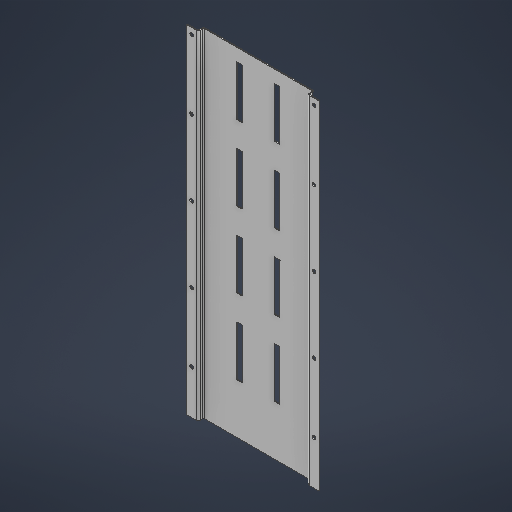
# Autodesk Inventor part: TrayRail
Saved by Autodesk Inventor 2026.3 (Build 303398000, 398)
## iProperties
Created: 2026-05-01
Part Number: TrayRail
Material: Generic
Document SubType Name: Sheet Metal
Designer: frede
Density: 1 g/cm^3
Sheet Metal Rule: Default_mm
Appearance: Default
Author: frede
Autodesk Inventor part; units mm, degrees
ref_plane "YZ Plane" through (0, 0, 0) normal (1, 0, 0) x (0, 1, 0)
ref_plane "XZ Plane" through (0, 0, 0) normal (0, 1, 0) x (-1, 0, 0)
ref_plane "XY Plane" through (0, 0, 0) normal (0, 0, 1) x (1, 0, 0)
sketch "Sketch1" plane through (0, 0, 0) normal (0, 0, 1) x (1, 0, 0)
  line L0 (61, -189) -> (-61, -189)
  line L1 (-61, -189) -> (-61, 189)
  line L2 (-61, 189) -> (61, 189)
  line L3 (61, 189) -> (61, -189)
  line L4 (61, -189) -> (-61, 189) construction
  line L5 (-61, -189) -> (61, 189) construction
  point P0 (0, 0)
  dimension "d0" = 122
  dimension "d1" = 378
  measures "d0" distance of L1.end L2.end
  measures "d1" distance between parallel lines of L0 L2
extrude "Plate1" add sketch "Sketch1" along normal blind 1
sketch "Sketch3" plane through (-62, -189, 0) normal (1, 0, 0) x (0, 1, 0)
  line L0 (378, 0) -> (0, 0)
  line L1 (0, 0) -> (0, 6)
  line L2 (0, 6) -> (378, 6)
  line L3 (378, 6) -> (378, 0)
  constraints: 8 end point
edge flange "Flange1" height 6 angle 90 thickness 1 bend radius 1 thickness toward (1, 0, 0) relief tear relief width 1 relief depth 0.5 corner gap 1 corner form 0 edges at (-61, 0, 1) (61, 0, 1) wall of the first edge with corners at (-62, 189, 0) (-62, -189, 0) (-62, -189, 6) (-62, 189, 6)
bend "Bend1"
corner "Corner1"
sketch "Sketch4" plane through (0, 0, 1) normal (0, 0, 1) x (1, 0, 0)
  line L0 (60, -189) -> (-60, -189) projected
  line L1 (-60, 189) -> (60, 189) projected
  line L2 (60.25, 63) -> (-60.25, 63)
  line L3 (-60.25, 63) -> (-60.25, 189)
  line L4 (-60.25, 189) -> (60.25, 189)
  line L5 (60.25, 189) -> (60.25, 63)
  line L6 (60.25, 63) -> (-60.25, 189) construction
  line L7 (-60.25, 63) -> (60.25, 189) construction
  line L8 (-21, 189) -> (-21, -189)
  line L9 (21, 189) -> (21, -189)
  line L10 (-24.25, 174.5) -> (-24.25, 119.5)
  line L11 (-17.75, 174.5) -> (-17.75, 119.5)
  line L12 (17.75, 174.5) -> (17.75, 119.5)
  line L13 (24.25, 174.5) -> (24.25, 119.5)
  line L14 (-23.75, 175) -> (-18.25, 175)
  line L15 (18.25, 175) -> (23.75, 175)
  line L16 (-23.75, 119) -> (-18.25, 119)
  line L17 (18.25, 119) -> (23.75, 119)
  arc A0 (-23.75, 175) -> (-24.25, 174.5) centre (-23.75, 174.5) ccw
  arc A1 (-17.75, 174.5) -> (-18.25, 175) centre (-18.25, 174.5) ccw
  arc A2 (-18.25, 119) -> (-17.75, 119.5) centre (-18.25, 119.5) ccw
  arc A3 (-24.25, 119.5) -> (-23.75, 119) centre (-23.75, 119.5) ccw
  arc A4 (17.75, 119.5) -> (18.25, 119) centre (18.25, 119.5) ccw
  arc A5 (23.75, 119) -> (24.25, 119.5) centre (23.75, 119.5) ccw
  arc A6 (18.25, 175) -> (17.75, 174.5) centre (18.25, 174.5) ccw
  arc A7 (24.25, 174.5) -> (23.75, 175) centre (23.75, 174.5) ccw
  line L18 (-23.75, 91) -> (-18.25, 91)
  arc A8 (-17.75, 90.5) -> (-18.25, 91) centre (-18.25, 90.5) ccw
  line L19 (-17.75, 90.5) -> (-17.75, 35.5)
  arc A9 (-23.75, 91) -> (-24.25, 90.5) centre (-23.75, 90.5) ccw
  line L20 (-24.25, 90.5) -> (-24.25, 35.5)
  line L21 (-23.75, 35) -> (-18.25, 35)
  arc A10 (-24.25, 35.5) -> (-23.75, 35) centre (-23.75, 35.5) ccw
  arc A11 (-18.25, 35) -> (-17.75, 35.5) centre (-18.25, 35.5) ccw
  line L22 (18.25, 35) -> (23.75, 35)
  arc A12 (23.75, 35) -> (24.25, 35.5) centre (23.75, 35.5) ccw
  arc A13 (17.75, 35.5) -> (18.25, 35) centre (18.25, 35.5) ccw
  line L23 (17.75, 90.5) -> (17.75, 35.5)
  line L24 (24.25, 90.5) -> (24.25, 35.5)
  line L25 (18.25, 91) -> (23.75, 91)
  arc A14 (24.25, 90.5) -> (23.75, 91) centre (23.75, 90.5) ccw
  arc A15 (18.25, 91) -> (17.75, 90.5) centre (18.25, 90.5) ccw
  line L26 (-23.75, 7) -> (-18.25, 7)
  arc A16 (-17.75, 6.5) -> (-18.25, 7) centre (-18.25, 6.5) ccw
  line L27 (-17.75, 6.5) -> (-17.75, -48.5)
  arc A17 (-23.75, 7) -> (-24.25, 6.5) centre (-23.75, 6.5) ccw
  line L28 (-24.25, 6.5) -> (-24.25, -48.5)
  line L29 (-23.75, -49) -> (-18.25, -49)
  arc A18 (-24.25, -48.5) -> (-23.75, -49) centre (-23.75, -48.5) ccw
  arc A19 (-18.25, -49) -> (-17.75, -48.5) centre (-18.25, -48.5) ccw
  line L30 (18.25, -49) -> (23.75, -49)
  arc A20 (23.75, -49) -> (24.25, -48.5) centre (23.75, -48.5) ccw
  arc A21 (17.75, -48.5) -> (18.25, -49) centre (18.25, -48.5) ccw
  line L31 (17.75, 6.5) -> (17.75, -48.5)
  line L32 (24.25, 6.5) -> (24.25, -48.5)
  line L33 (18.25, 7) -> (23.75, 7)
  arc A22 (24.25, 6.5) -> (23.75, 7) centre (23.75, 6.5) ccw
  arc A23 (18.25, 7) -> (17.75, 6.5) centre (18.25, 6.5) ccw
  line L34 (-23.75, -77) -> (-18.25, -77)
  arc A24 (-17.75, -77.5) -> (-18.25, -77) centre (-18.25, -77.5) ccw
  line L35 (-17.75, -77.5) -> (-17.75, -132.5)
  arc A25 (-23.75, -77) -> (-24.25, -77.5) centre (-23.75, -77.5) ccw
  line L36 (-24.25, -77.5) -> (-24.25, -132.5)
  line L37 (-23.75, -133) -> (-18.25, -133)
  arc A26 (-24.25, -132.5) -> (-23.75, -133) centre (-23.75, -132.5) ccw
  arc A27 (-18.25, -133) -> (-17.75, -132.5) centre (-18.25, -132.5) ccw
  line L38 (18.25, -133) -> (23.75, -133)
  arc A28 (23.75, -133) -> (24.25, -132.5) centre (23.75, -132.5) ccw
  arc A29 (17.75, -132.5) -> (18.25, -133) centre (18.25, -132.5) ccw
  line L39 (17.75, -77.5) -> (17.75, -132.5)
  line L40 (24.25, -77.5) -> (24.25, -132.5)
  line L41 (18.25, -77) -> (23.75, -77)
  arc A30 (24.25, -77.5) -> (23.75, -77) centre (23.75, -77.5) ccw
  arc A31 (18.25, -77) -> (17.75, -77.5) centre (18.25, -77.5) ccw
  line L42 (60.25, -63) -> (-60.25, -63)
  point P0 (0, 0)
  point P1 (0, 126)
  dimension "d17" = 120.5
  dimension "d18" = 60.25
  dimension "d19" = 21
  dimension "d20" = 42
  dimension "d22" = 6.5
  dimension "d23" = 3.25
  dimension "d24" = 6.5
  dimension "d25" = 3.25
  dimension "d26" = 56
  dimension "d27" = 56
  dimension "d28" = 0.5
  dimension "d31" = 84
  dimension "d38" = 126
  constraints: 82 end point, 64 point on circle, 32 centre point, 16 tangent, 7 equal radius, 7 perpendicular, 5 point on line, 4 vertical, 3 horizontal, 2 midpoint, 2 parallel, 123 other
  measures "d17" distance of L3.end L4.end
  measures "d18" distance from line of L3 point (0, 0)
  measures "d19" distance from line of point (0, 0) L8
  measures "d20" distance between parallel lines of L9 L8
  measures "d22" distance between parallel lines of L11 L10
  measures "d23" distance between parallel lines of L8 L10
  measures "d24" distance between parallel lines of L13 L12
  measures "d25" distance between parallel lines of L13 L9
  measures "d26" distance between parallel lines of L16 L14
  measures "d27" distance between parallel lines of L17 L15
  measures "d28" radius of A0
  measures "d31" distance of L14.start L18.start
  measures "d38" distance of L2.start L42.start
extrude "Extrusion2" cut sketch "Sketch4" against normal blind 2 contours L38 A29 L39 A31 L41 L9 | L9 L41 A30 L40 A28 L38 | L37 A26 L36 A25 L34 L8 | L8 L34 A24 L35 A27 L37 | L30 A21 L31 A23 L33 L9 | L9 L33 A22 L32 A20 L30 | L29 A18 L28 A17 L26 L8 | L8 L26 A16 L27 A19 L29 | L22 A13 L23 L2 L9 | L9 L2 L24 A12 L22 | L21 A10 L20 L2 L8 | L8 L2 L19 A11 L21 | L9 L25 A14 L24 L2 | L2 L23 A15 L25 L9 | L8 L18 A8 L19 L2 | L2 L20 A9 L18 L8 | L17 A4 L12 A6 L15 L9 | L9 L15 A7 L13 A5 L17 | L16 A3 L10 A0 L14 L8 | L8 L14 A1 L11 A2 L16
sketch "Sketch5" plane through (-61, 189, 7) normal (0, 0, -1) x (-1, 0, 0)
  line L0 (0, -378) -> (0, 0)
  line L1 (0, 0) -> (13, 0)
  line L2 (13, 0) -> (13, -378)
  line L3 (13, -378) -> (0, -378)
  constraints: 8 end point
edge flange "Flange2" height 13 angle 90 thickness 1 bend radius 1 thickness toward (0, 0, -1) relief tear relief width 1 relief depth 0.5 corner gap 1 corner form 0 edges at (-62, 0, 6) (62, 0, 6) wall of the first edge with corners at (-61, -189, 7) (-61, 189, 7) (-74, 189, 7) (-74, -189, 7)
bend "Bend2"
corner "Corner2"
sketch "Sketch7" plane through (-74, -189, 7) normal (0, 0, 1) x (1, 0, 0)
  line L0 (148, 378) -> (148, 0) projected
  line L1 (0, 0) -> (0, 378) projected
  line L2 (134, 0) -> (14, 0) projected
  line L3 (14, 378) -> (134, 378) projected
  line L4 (0, 364) -> (148, 364)
  line L5 (0, 308) -> (148, 308)
  line L6 (0, 280) -> (148, 280)
  line L7 (0, 224) -> (148, 224)
  line L8 (0, 196) -> (148, 196)
  line L9 (0, 140) -> (148, 140)
  line L10 (0, 112) -> (148, 112)
  line L11 (11, 378) -> (11, 0) projected
  line L12 (11, 308) -> (0, 280)
  line L13 (148, 308) -> (137, 280)
  line L14 (148, 224) -> (137, 196)
  line L15 (0, 196) -> (11, 224)
  line L16 (11, 140) -> (0, 112)
  line L17 (148, 140) -> (137, 112)
  line L18 (0, 364) -> (11, 378)
  line L19 (137, 364) -> (148, 378)
  line L20 (55.75, 56) -> (50.25, 56) projected
  line L21 (148, 56) -> (0, 56)
  line L22 (0, 42) -> (148, 42)
  line L23 (0, 42) -> (11, 56)
  line L24 (137, 42) -> (148, 56)
  point P0 (74, 189)
  point P1 (5.5, 294)
  point P2 (142.5, 294)
  point P3 (142.5, 210)
  point P4 (5.5, 210)
  point P5 (5.5, 126)
  point P6 (142.5, 126)
  point P7 (5.5, 49)
  point P8 (142.5, 49)
  point P9 (5.5, 371)
  point P10 (142.5, 371)
  dimension "d55" = 148
  dimension "d56" = 378
  dimension "d57" = 14
  constraints: 38 end point, 10 midpoint, 10 point on line, 9 horizontal, 7 parallel, 20 other
  measures "d56" distance between parallel lines of L2 L3
  measures "d57" distance between parallel lines of L22 L21
hole "Hole1" at (-68.5, 105, 7) at (68.5, 105, 7) at (68.5, 21, 7) at (-68.5, 21, 7) at (-68.5, -63, 7) at (68.5, -63, 7) at (-68.5, -140, 7) at (68.5, -140, 7) at (-68.5, 182, 7) at (68.5, 182, 7) direction (0, 0, -1) diameter 4 end through all
sketch "Sketch8" plane through (0, 0, 1) normal (0, 0, 1) x (1, 0, 0)
  line L0 (-23.75, 175) -> (-18.25, 175) projected
  circle A0 centre (-68.5, 182) radius 2 projected
  circle A1 centre (-68.5, 105) radius 2 projected
  line L1 (-23.75, 91) -> (-18.25, 91) projected
  line L2 (-23.75, 7) -> (-18.25, 7) projected
  circle A2 centre (-68.5, 21) radius 2 projected
  circle A3 centre (-68.5, -63) radius 2 projected
  line L3 (-23.75, -77) -> (-18.25, -77) projected
  circle A4 centre (-68.5, -140) radius 2 projected
  line L4 (-18.25, -133) -> (-23.75, -133) projected
  line L5 (-18.25, 35) -> (-23.75, 35) projected
  point P0 (0, 0)
  point P1 (-21, 35)
  dimension "d65" = 7
  dimension "d66" = 14
  dimension "d67" = 14
  dimension "d68" = 14
  dimension "d69" = 7
  dimension "d70" = 14
  constraints: 1 midpoint
  measures "d65" distance from line of L0 A0.centre
  measures "d66" distance from line of A1.centre L1
  measures "d67" distance from line of L2 A2.centre
  measures "d68" distance from line of A3.centre L3
  measures "d69" distance from line of A4.centre L4
  measures "d70" vertical distance of A2.centre point (-21, 35)
equation "\"d18\" = 0.5 * d17"
equation "\"d19\" = 0.5 * d20"
equation "\"d23\" = 0.5 * d22"
equation "\"d24\" = d22"
equation "\"d25\" = 0.5 * d24"
equation "\"d27\" = d26"
equation "\"d63\" = Thickness"
equation "\"d4\" = Thickness"
equation "\"d5\" = BendReliefWidth"
equation "\"d6\" = BendReliefDepth"
equation "\"d7\" = MinimumRemnant"
equation "\"d8\" = TransitionRadius"
equation "\"d11\" = BendRadius"
equation "\"d12\" = CornerReliefSize"
equation "\"d13\" = GapSize"
equation "\"d14\" = JacobiRadiusSize"
equation "\"d45\" = BendReliefWidth"
equation "\"d46\" = BendReliefDepth"
equation "\"d47\" = MinimumRemnant"
equation "\"d48\" = TransitionRadius"
equation "\"d51\" = BendRadius"
equation "\"d52\" = CornerReliefSize"
equation "\"d53\" = GapSize"
equation "\"d54\" = JacobiRadiusSize"
equation "\"BendRadius\" = Thickness"
equation "\"BendReliefWidth\" = Thickness"
equation "\"BendReliefDepth\" = 0.5 * Thickness"
equation "\"CornerReliefSize\" = 4 * Thickness"
equation "\"MinimumRemnant\" = 2 * Thickness"
equation "\"TransitionRadius\" = BendRadius"
equation "\"JacobiRadiusSize\" = BendRadius"
equation "\"GapSize\" = Thickness"
equation "\"Thickness\" = 1"
body "Solid2"
